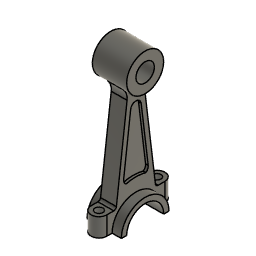
Connecting Rod (Autodesk Fusion 360 design; units mm, degrees)
Autodesk Fusion 360 part; units mm, degrees
note: some values were not read from the file. Chosen so that the rebuilt part matches the saved one: which face or edge a step refers to.
sketch "Sketch1" plane through (0, 0, 0) normal (1, 0, 0) x (0, 1, 0)
  arc A0 (177.8, 0) -> (-177.8, 0) centre (0, 0) ccw
  arc A1 (228.6, 0) -> (-228.6, 0) centre (0, 0) ccw
  line L0 (-177.8, 0) -> (-228.6, 0)
  line L1 (177.8, 0) -> (228.6, 0)
  dimension "d1" = 177.8
  dimension "d2" = 50.8
  constraint coincident A0.centre A1.centre
  constraint horizontal L0
  constraint horizontal L1
  constraint horizontal A0.centre A0.start
  measures "d1" radius of A0
extrude "Extrude1" add sketch "Sketch1" along normal mid plane 330.2
sketch "Sketch2" plane through (0, 0, 0) normal (1, 0, 0) x (0, 1, 0)
  line L0 (0, 0) -> (0, 1325.1758) construction
  arc A0 (228.6, 0) -> (-228.6, 0) centre (0, 0) ccw
  line L1 (-228.6, 0) -> (-355.6, 0)
  line L2 (-355.6, 0) -> (-355.6, 177.8)
  line L3 (-355.6, 177.8) -> (-190.5, 177.8)
  line L4 (-190.5, 177.8) -> (-76.1237, 1109.3201)
  line L5 (190.5, 177.8) -> (76.1237, 1109.3201)
  line L6 (355.6, 177.8) -> (190.5, 177.8)
  line L7 (355.6, 0) -> (355.6, 177.8)
  line L8 (355.6, 0) -> (228.6, 0)
  arc A1 (-76.1237, 1109.3201) -> (76.1237, 1109.3201) centre (0, 1270) ccw
  dimension "d5" = 355.6
  dimension "d6" = 1270
  dimension "d7" = 177.8
  dimension "d8" = 97
  dimension "d9" = 165.1
  dimension "d10" = 355.6
  constraint coincident L0.start A0.centre
  constraint vertical L0
  constraint coincident L0 A1.centre
  constraint coincident A0.end L1.start
  constraint horizontal L1
  constraint perpendicular L1 L2
  constraint perpendicular L2 L3
  constraint symmetric L0 L1.end L7.start
  constraint symmetric L0 L2.end L6.start
  constraint symmetric L0 L3.end L5.start
  constraint symmetric L0 L4.end L5.end
  constraint coincident A0.start L8.end
  measures "d5" diameter of A1
  measures "d6" distance of L0.start A1.centre
  measures "d7" distance of L1.end L2.end
  measures "d8" angle of L3 L4
  measures "d9" distance of L2.end L3.end
  measures "d10" distance of L0.start L2
extrude "Extrude2" add sketch "Sketch2" along normal mid plane 152.4
fillet "Fillet1" radius 76.2 2 edges at (-76.2, -355.6, 88.9) (76.2, -355.6, 88.9)
fillet "Fillet1" radius 76.2 2 edges at (-76.2, 355.6, 88.9) (76.2, 355.6, 88.9)
sketch "Sketch3" plane through (0, 0, 177.8) normal (0, 0, 1) x (-1, 0, 0)
  arc A0 (76.2, 279.4) -> (-76.2, 279.4) centre (0, 279.4) ccw
  line L0 (-76.2, 279.4) -> (-76.2, 190.5)
  line L1 (-76.2, 190.5) -> (76.2, 190.5)
  line L2 (76.2, 190.5) -> (76.2, 279.4)
  circle A1 centre (0, 279.4) radius 38.1
  circle A2 centre (0, -279.4) radius 38.1
  arc A3 (-76.2, -279.4) -> (76.2, -279.4) centre (0, -279.4) ccw
  dimension "d13" = 76.2
  dimension "d14" = 76.2
  constraint concentric A0 A1
  constraint concentric A2 A3
  measures "d13" diameter of A1
  measures "d14" diameter of A2
extrude "Extrude3" cut sketch "Sketch3" against normal blind 355.6 contours A1 | A2
sketch "Sketch4" plane through (0, 0, 0) normal (1, 0, 0) x (0, 1, 0)
  circle A0 centre (0, 1270) radius 177.8
  circle A1 centre (0, 1270) radius 88.9
  arc A2 (-76.1237, 1109.3201) -> (76.1237, 1109.3201) centre (0, 1270) ccw
  dimension "d17" = 355.6
  dimension "d18" = 177.8
  constraint concentric A0 A1
  constraint concentric A0 A2
  measures "d17" diameter of A0
  measures "d18" diameter of A1
extrude "Extrude4" add sketch "Sketch4" along normal mid plane 330.2
fillet "Fillet2" radius 25.4 2 edges at (0, -190.5, 177.8) (0, 190.5, 177.8)
fillet "Fillet2" radius 127 2 edges at (0, 76.1237, 1109.3201) (0, -76.1237, 1109.3201)
sketch "Sketch5" plane through (76.2, 0, 0) normal (1, 0, 0) x (0, 1, 0)
  line L0 (279.4, 0) -> (279.4, 177.8)
  line L1 (279.4, 177.8) -> (212.972, 177.8)
  arc A0 (187.7613, 200.1045) -> (212.972, 177.8) centre (212.972, 203.2) ccw
  line L2 (187.7613, 200.1045) -> (85.2651, 1034.8694)
  arc A1 (123.2691, 1141.8689) -> (85.2651, 1034.8694) centre (211.3185, 1050.3468) ccw
  arc A2 (-123.2691, 1141.8689) -> (123.2691, 1141.8689) centre (0, 1270) ccw
  arc A3 (-85.2651, 1034.8694) -> (-123.2691, 1141.8689) centre (-211.3185, 1050.3468) ccw
  line L3 (-85.2651, 1034.8694) -> (-187.7613, 200.1045)
  arc A4 (-212.972, 177.8) -> (-187.7613, 200.1045) centre (-212.972, 203.2) ccw
  line L4 (-212.972, 177.8) -> (-279.4, 177.8)
  line L5 (-279.4, 177.8) -> (-279.4, 0)
  line L6 (-279.4, 0) -> (-228.6, 0)
  arc A5 (228.6, 0) -> (-228.6, 0) centre (0, 0) ccw
  line L7 (228.6, 0) -> (279.4, 0)
  arc A6 (-118.2931, 390.7218) -> (-96.1766, 342.3469) centre (-67.8718, 384.5308) ccw
  line L8 (-118.2931, 390.7218) -> (-50.4213, 943.4932)
  arc A7 (50.4213, 943.4932) -> (-50.4213, 943.4932) centre (0, 937.3023) ccw
  line L9 (50.4213, 943.4932) -> (118.2931, 390.7218)
  arc A8 (96.1766, 342.3469) -> (118.2931, 390.7218) centre (67.8718, 384.5308) ccw
  arc A9 (96.1766, 342.3469) -> (-96.1766, 342.3469) centre (0, 0) ccw
  dimension "d25" = 711.2
  dimension "d26" = 50.8
  dimension "d27" = 45.72
  dimension "d28" = 45.72
  dimension "d29" = 50.8
  dimension "d30" = 50.8
  constraint concentric A5 A9
  constraint parallel L3 L8
  constraint tangent L8 A7
  constraint tangent L9 A8
  constraint parallel L2 L9
  constraint tangent A6 L8
  constraint equal L8 L9
  constraint tangent A7 L9
  measures "d25" diameter of A9
  measures "d26" radius of A7
  measures "d27" distance of L3 L8
  measures "d28" distance of L2 L9
  measures "d29" radius of A8
  measures "d30" radius of A6
extrude "Extrude5" cut sketch "Sketch5" against normal blind 25.4 contours A6 L8 A7 L9 A8 A9
mirror "Mirror1" about plane through (0, 0, 0) normal (1, 0, 0) of "Extrude5"
